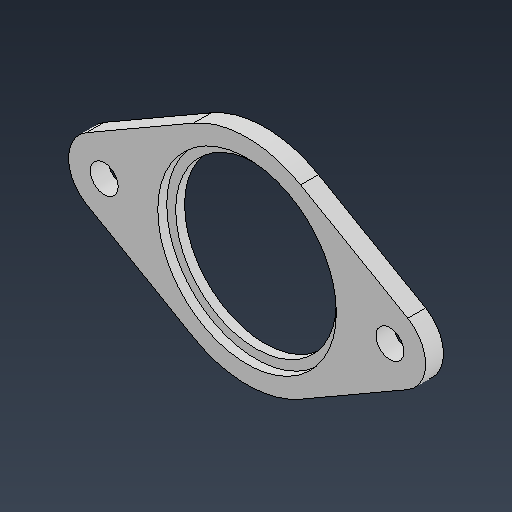
# Autodesk Inventor part: Bearing Holder
Saved by Autodesk Inventor 2026 (Build 300175050, 175E)
## iProperties
Created: 2026-01-18
Part Number: Bearing Holder
Material: Generic
Document SubType Name: Modeling
Designer: Jthib
Mass: 2.62409 g
Surface Area: 26.9406 cm^2
Volume: 2.62409 cm^3
Density: 1 g/cm^3
Appearance: Default
Author: Jthib
Autodesk Inventor part; units mm, degrees
ref_plane "YZ Plane" through (0, 0, 0) normal (1, 0, 0) x (0, 1, 0)
ref_plane "XZ Plane" through (0, 0, 0) normal (0, 1, 0) x (-1, 0, 0)
ref_plane "XY Plane" through (0, 0, 0) normal (0, 0, 1) x (1, 0, 0)
sketch "Sketch1" plane through (0, 0, 0) normal (0, 0, 1) x (1, 0, 0)
  line L0 (-9.525, 16.4978) -> (-28.575, 5.4993)
  arc A0 (-28.575, 5.4993) -> (-28.575, -5.4993) centre (-25.4, 0) ccw
  line L1 (-28.575, -5.4993) -> (-9.525, -16.4978)
  line L2 (9.525, 16.4978) -> (28.575, 5.4993)
  arc A1 (28.575, -5.4993) -> (28.575, 5.4993) centre (25.4, 0) ccw
  line L3 (28.575, -5.4993) -> (9.525, -16.4978)
  arc A2 (-9.525, -16.4978) -> (9.525, -16.4978) centre (0, 0) ccw
  arc A3 (9.525, 16.4978) -> (-9.525, 16.4978) centre (0, 0) ccw
  line L4 (-44.45, 0) -> (44.45, 0) construction
  line L5 (0, -26.67) -> (0, 26.67) construction
  dimension "d0" = 6.35
  dimension "d1" = 50.8
  dimension "d2" = 19.05
  constraints: 8 end point, 8 point on circle, 8 tangent, 4 centre point, 2 equal length, 2 equal radius, 2 point on line, 1 coincident
  measures "d0" radius of A0
  measures "d1" distance of A1.centre A0.centre
  measures "d2" radius of A3
extrude "Extrusion1" add sketch "Sketch1" along normal blind 3.175
sketch "Sketch2" plane through (0, 0, 3.175) normal (0, 0, 1) x (1, 0, 0)
  point P0 (0, 0)
hole "Hole1" at (0, 0, 3.175) direction (0, 0, -1) diameter 28.575 end through all counterbore diameter 31.75 counterbore depth 1.5875
sketch "Sketch3" plane through (0, 0, 3.175) normal (0, 0, 1) x (1, 0, 0)
  arc A0 (-28.575, 5.4993) -> (-28.575, -5.4993) centre (-25.4, 0) ccw construction
  arc A1 (28.575, -5.4993) -> (28.575, 5.4993) centre (25.4, 0) ccw construction
  point P0 (0, 0)
  point P1 (-25.4, 0)
  constraints: 2 coincident
hole "Hole2" at (-25.4, 0, 3.175) at (25.4, 0, 3.175) direction (0, 0, -1) diameter 4.9784 end through all clearance for "Flat Head Machine Screw (82)" size "#10" standard "Ansi Unified Screw Threads"
body "Solid1"
